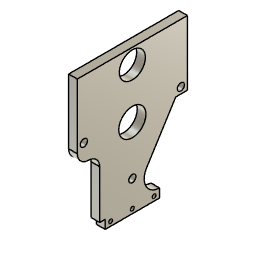
[J,L]C-578VA Mount (Autodesk Fusion 360 design; units mm, degrees)
Autodesk Fusion 360 part; units mm, degrees
sketch "スケッチ1" plane through (0, 0, 0) normal (1, 0, 0) x (0, 1, 0)
  line L0 (0, 0) -> (-44.6, 0)
  line L1 (0, 0) -> (44.6, 0)
  line L2 (-44.6, 0) -> (-44.6, 5.7)
  line L3 (44.6, 0) -> (44.6, 5.7)
  circle A0 centre (-44.6, 5.7) radius 3
  circle A1 centre (44.6, 5.7) radius 3
  line L4 (0, 0) -> (0, 43.5)
  line L5 (0, 43.5) -> (-11.3, 43.5)
  circle A2 centre (-11.3, 43.5) radius 3
  line L6 (0, 0) -> (0, -45)
  circle A3 centre (0, -45) radius 3
  circle A4 centre (-11.3, 43.5) radius 6
  circle A5 centre (-44.6, 5.7) radius 6
  circle A6 centre (44.6, 5.7) radius 6
  circle A7 centre (0, -45) radius 6
  line L7 (50.6, -51) -> (-50.6, -51)
  line L8 (-50.6, -51) -> (-50.6, 51)
  line L9 (-50.6, 51) -> (50.6, 51)
  line L10 (50.6, 51) -> (50.6, -51)
  line L11 (50.6, -51) -> (-50.6, 51) construction
  line L12 (-50.6, -51) -> (50.6, 51) construction
  circle A8 centre (0, 0) radius 10.5
  line L13 (44.6, 5.7) -> (0, -45)
  line L14 (44.6, 5.7) -> (50.6, 5.7) construction
  line L15 (0, -45) -> (4.505, -48.963)
  line L16 (44.6, 5.7) -> (49.105, 1.737)
  line L17 (0, -45) -> (6, -45)
  line L18 (44.6, 5.7) -> (44.6, -0.3)
  dimension "d1" = 44.6
  dimension "d2" = 44.6
  dimension "d3" = 5.7
  dimension "d4" = 5.7
  dimension "d5" = 6
  dimension "d6" = 6
  dimension "d7" = 43.5
  dimension "d8" = 11.3
  dimension "d9" = 6
  dimension "d10" = 45
  dimension "d11" = 6
  dimension "d12" = 12
  dimension "d13" = 12
  dimension "d14" = 12
  dimension "d15" = 12
  dimension "d16" = 101.2
  dimension "d17" = 102
  dimension "d20" = 21
  constraint coincident L0.start L1.start
  constraint horizontal L0
  constraint parallel L0 L1
  constraint perpendicular L0 L2
  constraint perpendicular L1 L3
  constraint coincident L2.end A0.centre
  constraint coincident L3.end A1.centre
  constraint perpendicular L1 L4
  constraint perpendicular L4 L5
  constraint coincident L5.end A2.centre
  constraint perpendicular L1 L6
  constraint coincident L6.end A3.centre
  constraint concentric A2 A4
  constraint concentric A0 A5
  constraint concentric A1 A6
  constraint concentric A3 A7
  constraint horizontal L7
  constraint perpendicular L7 L8
  constraint parallel L7 L9
  constraint parallel L8 L10
  constraint coincident L11 L0.start
  constraint coincident L12 L0.start
  constraint horizontal L14
  constraint coincident A7 L15.end
  constraint perpendicular L13 L15
  constraint coincident A6 L16.end
  constraint perpendicular L13 L16
  constraint coincident A7 L17.end
  constraint perpendicular L6 L17
  constraint coincident A6 L18.end
  constraint perpendicular L14 L18
  measures "d1" distance of L0.start L0.end
  measures "d2" distance of L0.start L1.end
  measures "d3" distance of L0.end L2.end
  measures "d4" distance of L1.end L3.end
  measures "d5" diameter of A0
  measures "d6" diameter of A1
  measures "d7" distance of L0.start L4.end
  measures "d8" distance of L4.end L5.end
  measures "d9" diameter of A2
  measures "d10" distance of L0.start L6.end
  measures "d11" diameter of A3
  measures "d12" diameter of A4
  measures "d13" diameter of A5
  measures "d14" diameter of A6
  measures "d15" diameter of A7
  measures "d16" distance of L8.end L9.end
  measures "d17" distance of L7.end L8.end
  measures "d20" diameter of A8
extrude "押し出し1" add sketch "スケッチ1" along normal blind 8 contours L0 L6 A5 A7 L7 L8 A8 | L0 L1 A5 A6 L8 L9 L10 A8 L13 | L1 L6 A7 A8 L13 | A5 | L6 A3 A7 L13 | L6 A3 A7 L15 | L1 L3 A1 A6 L13 L18 | L1 A6 L18 | A1 A6 L13 L16 | A3 A7 L13 L17 | L3 A1 A6 L16 L18 | A3 A7 L15 L17 | A4
sketch "スケッチ2" plane through (0, 0, -51) normal (0, 0, -1) x (1, 0, 0)
  line L0 (0, 50.6) -> (0, 0)
  line L1 (0, 0) -> (8, 0)
  line L2 (8, 0) -> (8, 50.6)
  line L3 (8, 50.6) -> (0, 50.6)
  line L4 (0, 50.6) -> (8, 50.6)
  line L5 (8, 50.6) -> (8, 0.6)
  line L6 (8, 0.6) -> (0, 0.6)
  line L7 (0, 0.6) -> (0, 50.6)
  dimension "d22" = 50
  constraint horizontal L4
  constraint vertical L5
  constraint horizontal L6
  constraint vertical L7
  constraint coincident L0.start L3.end
  measures "d22" distance of L0.start L6.end
extrude "押し出し2" add sketch "スケッチ2" along normal blind 18 contours L0 L2 L3 L4 L5 L6 L7
sketch "スケッチ3" plane through (0, 0, 0) normal (-1, 0, 0) x (0, -1, 0)
  circle A0 centre (11.3, 43.5) radius 3
  circle A1 centre (44.6, 5.7) radius 3
  circle A2 centre (0, 0) radius 10.5
  circle A3 centre (-44.6, 5.7) radius 3
  circle A4 centre (0, -45) radius 3
  arc A5 (-3.963, -40.495) -> (0, -51) centre (0, -45) ccw
  line L0 (0, -51) -> (0.6, -51)
  line L1 (0.6, -51) -> (0.6, -69)
  line L2 (0.6, -69) -> (50.6, -69)
  line L3 (50.6, -69) -> (50.6, 51)
  line L4 (50.6, 51) -> (-50.6, 51)
  line L5 (-50.6, 51) -> (-50.6, 5.7)
  arc A6 (-50.6, 5.7) -> (-40.637, 1.195) centre (-44.6, 5.7) ccw
  line L6 (-40.637, 1.195) -> (-3.963, -40.495)
  circle A7 centre (0, 0) radius 23.5
  dimension "d25" = 47
  constraint coincident A2.centre A7.centre
  measures "d25" diameter of A7
extrude "押し出し3" cut sketch "スケッチ3" against normal blind 8 contours A7
extrude "押し出し4" add 1 faces at (2.6667, -17.2667, -69) along direction (0, 0, -1) blind 4
box "直方体プリミティブ1" cut length 8 width 8 height -25.6 placed x (0, 0, 1) y (-1, 0, 0) z (0, -1, 0) at (8, -50.6, -73)
box "直方体プリミティブ2" add length 8 width 8 height 25.6 placed x (0, 0, 1) y (1, 0, 0) z (0, 1, 0) at (0, -0.6, -73)
sketch "スケッチ7" plane through (0, 0, 0) normal (-1, 0, 0) x (0, -1, 0)
  line L0 (25, -73) -> (25, -65)
  line L1 (25, -65) -> (50.6, -65)
  line L2 (50.6, -65) -> (50.6, 51)
  line L3 (50.6, 51) -> (-50.6, 51)
  line L4 (-50.6, 51) -> (-50.6, 5.7)
  arc A0 (-50.6, 5.7) -> (-40.637, 1.195) centre (-44.6, 5.7) ccw
  line L5 (-40.637, 1.195) -> (-3.963, -40.495)
  arc A1 (-3.963, -40.495) -> (0, -51) centre (0, -45) ccw
  line L6 (0, -51) -> (0.6, -51)
  line L7 (0.6, -51) -> (0.6, -65)
  line L8 (0.6, -65) -> (-25, -65)
  line L9 (-25, -65) -> (-25, -73)
  line L10 (-25, -73) -> (25, -73)
  circle A2 centre (0, -45) radius 3
  circle A3 centre (-44.6, 5.7) radius 3
  circle A4 centre (44.6, 5.7) radius 3
  circle A5 centre (11.3, 43.5) radius 3
  circle A6 centre (0, 0) radius 23.5
  line L11 (25, -65) -> (30, -65)
  line L12 (0, 0) -> (0, -23.5)
  line L13 (0, -23.5) -> (50.6, -23.5)
  line L14 (30, -65) -> (30, -23.5)
  dimension "d48" = 5
  constraint coincident L0.end L1.start
  constraint perpendicular L0 L11
  constraint coincident A6.centre L12.start
  constraint coincident A6 L12.end
  constraint vertical L12
  constraint coincident L2 L13.end
  constraint tangent A6 L13
  constraint coincident L13 L14.end
  constraint perpendicular L13 L14
  measures "d48" distance of L0.end L11.end
extrude "押し出し6" cut sketch "スケッチ7" against normal blind 8 contours L1 L2 L13 L14
extrude "押し出し7" cut 1 faces at (2.6667, -36.8667, -23.5) along direction (0, 0, 1) blind 5
sketch "スケッチ8" plane through (8, 0, 0) normal (1, 0, 0) x (0, 1, 0)
  line L0 (-50.6, -18.5) -> (-30, -18.5)
  line L1 (-30, -18.5) -> (-30, -65)
  line L2 (-30, -65) -> (-25, -65)
  line L3 (-25, -65) -> (-25, -73)
  line L4 (-25, -73) -> (25, -73)
  line L5 (25, -73) -> (25, -65)
  line L6 (25, -65) -> (-0.6, -65)
  line L7 (-0.6, -65) -> (-0.6, -51)
  line L8 (-0.6, -51) -> (0, -51)
  arc A0 (0, -51) -> (3.963, -40.495) centre (0, -45) ccw
  line L9 (3.963, -40.495) -> (40.637, 1.195)
  arc A1 (40.637, 1.195) -> (50.6, 5.7) centre (44.6, 5.7) ccw
  line L10 (50.6, 5.7) -> (50.6, 51)
  line L11 (50.6, 51) -> (-50.6, 51)
  line L12 (-50.6, 51) -> (-50.6, -18.5)
  circle A2 centre (0, -45) radius 3
  circle A3 centre (44.6, 5.7) radius 3
  circle A4 centre (-44.6, 5.7) radius 3
  circle A5 centre (-11.3, 43.5) radius 3
  circle A6 centre (0, 0) radius 23.5
  line L13 (40.637, 1.195) -> (-0.6, -65)
  constraint coincident L9.end A1.start
  constraint coincident L6.end L7.start
extrude "押し出し8" add sketch "スケッチ8" against normal blind 8 contours L7 L8 A0 L9 L13
fillet "フィレット1" radius 14.3 1 edges at (4, -0.6, -65)
fillet "フィレット2" radius 10.3 1 edges at (4, -50.6, -18.5)
fillet "フィレット3" radius 10.3 1 edges at (4, -30, -18.5)
sketch "スケッチ9" plane through (8, 0, 0) normal (1, 0, 0) x (0, 1, 0)
  arc A0 (-50.6, -8.2) -> (-40.3, -18.5) centre (-40.3, -8.2) ccw
  arc A1 (-30, -28.8) -> (-40.3, -18.5) centre (-40.3, -28.8) ccw
  line L0 (-30, -28.8) -> (-30, -65)
  line L1 (-30, -65) -> (-25, -65)
  line L2 (-25, -65) -> (-25, -73)
  line L3 (-25, -73) -> (25, -73)
  line L4 (25, -73) -> (25, -65)
  arc A2 (13.0182, -43.1397) -> (25, -65) centre (25.1557, -50.7008) ccw
  line L5 (13.0182, -43.1397) -> (40.637, 1.195)
  arc A3 (40.637, 1.195) -> (50.6, 5.7) centre (44.6, 5.7) ccw
  line L6 (50.6, 5.7) -> (50.6, 51)
  line L7 (50.6, 51) -> (-50.6, 51)
  line L8 (-50.6, 51) -> (-50.6, -8.2)
  circle A4 centre (0, -45) radius 3
  circle A5 centre (44.6, 5.7) radius 3
  circle A6 centre (-44.6, 5.7) radius 3
  circle A7 centre (-11.3, 43.5) radius 3
  circle A8 centre (0, 0) radius 23.5
  line L9 (-25, -69) -> (25, -69)
  line L10 (0, -69) -> (20, -69)
  line L11 (0, -69) -> (-20, -69)
  circle A9 centre (0, -69) radius 1.7
  circle A10 centre (-20, -69) radius 1.7
  circle A11 centre (20, -69) radius 1.7
  dimension "d61" = 20
  dimension "d62" = 20
  dimension "d63" = 3.4
  dimension "d64" = 3.4
  dimension "d65" = 3.4
  constraint midpoint L2 L9.start
  constraint midpoint L4 L9.end
  constraint midpoint L9 L10.start
  constraint perpendicular L4 L10
  constraint parallel L9 L11
  constraint coincident L10.start L11.start
  constraint coincident L11.end A10.centre
  constraint coincident L10.end A11.centre
  measures "d61" distance of L10.start L10.end
  measures "d62" distance of L10.start L11.end
  measures "d63" diameter of A9
  measures "d64" diameter of A10
  measures "d65" diameter of A11
extrude "押し出し9" cut sketch "スケッチ9" against normal blind 8 contours L9 L11 A10 | L9 L11 A10 | L9 L10 L11 A9 | L9 L10 L11 A9 | L9 L10 A11 | L9 L10 A11
sketch "スケッチ10" plane through (8, 0, 0) normal (1, 0, 0) x (0, 1, 0)
  circle A0 centre (20, -69) radius 1.7
  circle A1 centre (0, -69) radius 1.7
  circle A2 centre (-20, -69) radius 1.7
  arc A3 (-50.6, -8.2) -> (-40.3, -18.5) centre (-40.3, -8.2) ccw
  arc A4 (-30, -28.8) -> (-40.3, -18.5) centre (-40.3, -28.8) ccw
  line L0 (-30, -28.8) -> (-30, -65)
  line L1 (-30, -65) -> (-25, -65)
  line L2 (-25, -65) -> (-25, -73)
  line L3 (-25, -73) -> (25, -73)
  line L4 (25, -73) -> (25, -65)
  arc A5 (13.0182, -43.1397) -> (25, -65) centre (25.1557, -50.7008) ccw
  line L5 (13.0182, -43.1397) -> (40.637, 1.195)
  arc A6 (40.637, 1.195) -> (50.6, 5.7) centre (44.6, 5.7) ccw
  line L6 (50.6, 5.7) -> (50.6, 51)
  line L7 (50.6, 51) -> (-50.6, 51)
  line L8 (-50.6, 51) -> (-50.6, -8.2)
  circle A7 centre (0, -45) radius 3
  circle A8 centre (44.6, 5.7) radius 3
  circle A9 centre (-44.6, 5.7) radius 3
  circle A10 centre (-11.3, 43.5) radius 3
  circle A11 centre (0, 0) radius 23.5
  line L9 (0, 0) -> (0, 45.5)
  circle A12 centre (0, 45.5) radius 12
  line L10 (-50.6, 51) -> (0, 51)
  line L11 (0, 51) -> (0, 57.5)
  line L12 (0, 57.5) -> (-50.6, 57.5)
  line L13 (-50.6, 57.5) -> (-50.6, 51)
  line L14 (50.6, 51) -> (0, 51)
  line L15 (0, 51) -> (0, 57.5)
  line L16 (0, 57.5) -> (50.6, 57.5)
  line L17 (50.6, 57.5) -> (50.6, 51)
  line L18 (-50.6, 57.5) -> (50.6, 57.5)
  line L19 (50.6, 57.5) -> (50.6, 59.5)
  line L20 (50.6, 59.5) -> (-50.6, 59.5)
  line L21 (-50.6, 59.5) -> (-50.6, 57.5)
  dimension "d68" = 45.5
  dimension "d69" = 24
  dimension "d72" = 2
  constraint coincident A11.centre L9.start
  constraint vertical L9
  constraint coincident L9.end A12.centre
  constraint horizontal L10
  constraint vertical L11
  constraint horizontal L12
  constraint vertical L13
  constraint coincident A12 L11.end
  constraint coincident L7.end L8.start
  constraint horizontal L14
  constraint vertical L15
  constraint horizontal L16
  constraint vertical L17
  constraint coincident L6.end L7.start
  constraint horizontal L18
  constraint vertical L19
  constraint horizontal L20
  constraint vertical L21
  measures "d68" distance of A11.centre L9.end
  measures "d69" diameter of A12
  measures "d72" distance of L12.end L20.end
extrude "押し出し11" add sketch "スケッチ10" against normal blind 8 contours L7 A12 L10 L12 L13 L18 | L12 L16 L18 L19 L20 L21 | L7 A12 L14 L16 L17 L18
extrude "押し出し12" cut sketch "スケッチ10" against normal blind 8 contours L7 A10 A12 L10 L14
extrude "押し出し13" add sketch "スケッチ10" against normal blind 8 contours A10 A12 picked at (-12.6459, 44.2666)
sketch "スケッチ11" plane through (8, 0, 0) normal (1, 0, 0) x (0, 1, 0)
  circle A0 centre (0, 45.5) radius 12
  line L0 (-50.6, 59.5) -> (-50.6, -8.2)
  arc A1 (-50.6, -8.2) -> (-40.3, -18.5) centre (-40.3, -8.2) ccw
  arc A2 (-30, -28.8) -> (-40.3, -18.5) centre (-40.3, -28.8) ccw
  line L1 (-30, -28.8) -> (-30, -65)
  line L2 (-30, -65) -> (-25, -65)
  line L3 (-25, -65) -> (-25, -73)
  line L4 (-25, -73) -> (25, -73)
  line L5 (25, -73) -> (25, -65)
  arc A3 (13.0182, -43.1397) -> (25, -65) centre (25.1557, -50.7008) ccw
  line L6 (13.0182, -43.1397) -> (40.637, 1.195)
  arc A4 (40.637, 1.195) -> (50.6, 5.7) centre (44.6, 5.7) ccw
  line L7 (50.6, 5.7) -> (50.6, 59.5)
  line L8 (50.6, 59.5) -> (-50.6, 59.5)
  circle A5 centre (20, -69) radius 1.7
  circle A6 centre (0, -69) radius 1.7
  circle A7 centre (-20, -69) radius 1.7
  circle A8 centre (0, -45) radius 3
  circle A9 centre (44.6, 5.7) radius 3
  circle A10 centre (-44.6, 5.7) radius 3
  circle A11 centre (0, 0) radius 23.5
  circle A12 centre (0, 0) radius 13
  dimension "d79" = 26
  constraint coincident A11.centre A12.centre
  measures "d79" diameter of A12
extrude "押し出し14" add sketch "スケッチ11" against normal blind 8 contours A11
sketch "スケッチ12" plane through (8, 0, 0) normal (1, 0, 0) x (0, 1, 0)
  circle A0 centre (0, 0) radius 13
  circle A1 centre (0, 45.5) radius 12
  line L0 (-50.6, 59.5) -> (-50.6, -8.2)
  arc A2 (-50.6, -8.2) -> (-40.3, -18.5) centre (-40.3, -8.2) ccw
  arc A3 (-30, -28.8) -> (-40.3, -18.5) centre (-40.3, -28.8) ccw
  line L1 (-30, -28.8) -> (-30, -65)
  line L2 (-30, -65) -> (-25, -65)
  line L3 (-25, -65) -> (-25, -73)
  line L4 (-25, -73) -> (25, -73)
  line L5 (25, -73) -> (25, -65)
  arc A4 (13.0182, -43.1397) -> (25, -65) centre (25.1557, -50.7008) ccw
  line L6 (13.0182, -43.1397) -> (40.637, 1.195)
  arc A5 (40.637, 1.195) -> (50.6, 5.7) centre (44.6, 5.7) ccw
  line L7 (50.6, 5.7) -> (50.6, 59.5)
  line L8 (50.6, 59.5) -> (-50.6, 59.5)
  circle A6 centre (20, -69) radius 1.7
  circle A7 centre (0, -69) radius 1.7
  circle A8 centre (-20, -69) radius 1.7
  circle A9 centre (0, -45) radius 3
  circle A10 centre (44.6, 5.7) radius 3
  circle A11 centre (-44.6, 5.7) radius 3
  line L9 (44.6, 5.7) -> (44.6, -0.3)
  line L10 (44.6, -0.3) -> (39.7057, -0.3)
  constraint coincident A5.centre A10.centre
  constraint coincident A5 L9.end
  constraint vertical L9
  constraint coincident L6 L10.end
  constraint tangent A5 L10
extrude "押し出し15" add sketch "スケッチ12" against normal blind 8 contours L6 A5 L10
sketch "スケッチ13" plane through (8, 0, 0) normal (1, 0, 0) x (0, 1, 0)
  circle A0 centre (0, 0) radius 13
  circle A1 centre (0, 45.5) radius 12
  line L0 (-50.6, 59.5) -> (-50.6, -8.2)
  arc A2 (-50.6, -8.2) -> (-40.3, -18.5) centre (-40.3, -8.2) ccw
  arc A3 (-30, -28.8) -> (-40.3, -18.5) centre (-40.3, -28.8) ccw
  line L1 (-30, -28.8) -> (-30, -65)
  line L2 (-30, -65) -> (-25, -65)
  line L3 (-25, -65) -> (-25, -73)
  line L4 (-25, -73) -> (25, -73)
  line L5 (25, -73) -> (25, -65)
  arc A4 (13.0182, -43.1397) -> (25, -65) centre (25.1557, -50.7008) ccw
  line L6 (13.0182, -43.1397) -> (39.7057, -0.3)
  line L7 (39.7057, -0.3) -> (44.6, -0.3)
  arc A5 (44.6, -0.3) -> (50.6, 5.7) centre (44.6, 5.7) ccw
  line L8 (50.6, 5.7) -> (50.6, 59.5)
  line L9 (50.6, 59.5) -> (-50.6, 59.5)
  circle A6 centre (20, -69) radius 1.7
  circle A7 centre (0, -69) radius 1.7
  circle A8 centre (-20, -69) radius 1.7
  circle A9 centre (0, -45) radius 3
  circle A10 centre (44.6, 5.7) radius 3
  circle A11 centre (-44.6, 5.7) radius 3
  line L10 (0, 0) -> (-50.6, 0)
  line L11 (44.6, 5.7) -> (44.6, 0)
  line L12 (44.6, 0) -> (0, 0)
  line L13 (50.6, 5.7) -> (44.6, 5.7)
  line L14 (44.6, 5.7) -> (44.6, 0)
  line L15 (44.6, 0) -> (50.6, 0)
  line L16 (50.6, 0) -> (50.6, 5.7)
  constraint coincident A0.centre L10.start
  constraint coincident L0 L10.end
  constraint perpendicular L0 L10
  constraint coincident A5.centre A10.centre
  constraint perpendicular L10 L11
  constraint perpendicular L11 L12
  constraint horizontal L13
  constraint vertical L14
  constraint horizontal L15
  constraint vertical L16
  constraint coincident A5.end L8.start
extrude "押し出し17" add sketch "スケッチ13" against normal blind 8 contours A5 L15 L16
sketch "スケッチ14" plane through (8, 0, 0) normal (1, 0, 0) x (0, 1, 0)
  circle A0 centre (0, 0) radius 13
  circle A1 centre (0, 45.5) radius 12
  line L0 (-50.6, 59.5) -> (-50.6, -8.2)
  arc A2 (-50.6, -8.2) -> (-40.3, -18.5) centre (-40.3, -8.2) ccw
  arc A3 (-30, -28.8) -> (-40.3, -18.5) centre (-40.3, -28.8) ccw
  line L1 (-30, -28.8) -> (-30, -65)
  line L2 (-30, -65) -> (-25, -65)
  line L3 (-25, -65) -> (-25, -73)
  line L4 (-25, -73) -> (25, -73)
  line L5 (25, -73) -> (25, -65)
  arc A4 (13.0182, -43.1397) -> (25, -65) centre (25.1557, -50.7008) ccw
  line L6 (13.0182, -43.1397) -> (39.7057, -0.3)
  line L7 (39.7057, -0.3) -> (44.6, -0.3)
  arc A5 (44.6, -0.3) -> (46.4735, 0) centre (44.6, 5.7) ccw
  line L8 (46.4735, 0) -> (50.6, 0)
  line L9 (50.6, 0) -> (50.6, 59.5)
  line L10 (50.6, 59.5) -> (-50.6, 59.5)
  circle A6 centre (20, -69) radius 1.7
  circle A7 centre (0, -69) radius 1.7
  circle A8 centre (-20, -69) radius 1.7
  circle A9 centre (0, -45) radius 3
  circle A10 centre (44.6, 5.7) radius 3
  circle A11 centre (-44.6, 5.7) radius 3
  line L11 (0, 0) -> (46.4735, 0)
  line L12 (39.7057, -0.3) -> (39.8926, 0)
  constraint coincident A0.centre L11.start
  constraint coincident A5.end L8.start
  constraint coincident L6.end L7.start
  constraint coincident L11 L12.end
  constraint parallel L6 L12
extrude "押し出し18" cut sketch "スケッチ14" against normal blind 8 contours L7 A5 L11 L12
sketch "スケッチ15" plane through (8, 0, 0) normal (1, 0, 0) x (0, 1, 0)
  line L0 (39.8926, 0) -> (50.6, 0)
  line L1 (50.6, 0) -> (50.6, 59.5)
  line L2 (50.6, 59.5) -> (-50.6, 59.5)
  line L3 (-50.6, 59.5) -> (-50.6, -8.2)
  arc A0 (-50.6, -8.2) -> (-40.3, -18.5) centre (-40.3, -8.2) ccw
  arc A1 (-30, -28.8) -> (-40.3, -18.5) centre (-40.3, -28.8) ccw
  line L4 (-30, -28.8) -> (-30, -65)
  line L5 (-30, -65) -> (-25, -65)
  line L6 (-25, -65) -> (-25, -73)
  line L7 (-25, -73) -> (25, -73)
  line L8 (25, -73) -> (25, -65)
  arc A2 (13.0182, -43.1397) -> (25, -65) centre (25.1557, -50.7008) ccw
  line L9 (13.0182, -43.1397) -> (39.8926, 0)
  circle A3 centre (0, 0) radius 13
  circle A4 centre (0, 45.5) radius 12
  circle A5 centre (20, -69) radius 1.7
  circle A6 centre (0, -69) radius 1.7
  circle A7 centre (-20, -69) radius 1.7
  circle A8 centre (0, -45) radius 3
  circle A9 centre (44.6, 5.7) radius 3
  circle A10 centre (-44.6, 5.7) radius 3
  line L10 (0, 0) -> (-50.6, 0)
  line L11 (-40.3, -18.5) -> (-40.3, 0)
  circle A11 centre (-40.3, 0) radius 10.3
  line L12 (-40.3, -10.3) -> (-30, -10.3)
  line L13 (-30, -10.3) -> (-30, -20.6)
  line L14 (-30, -20.6) -> (-40.3, -20.6)
  line L15 (-40.3, -20.6) -> (-40.3, -10.3)
  circle A12 centre (-40.3, -20.6) radius 10.3
  line L16 (-30, -20.6) -> (-30, -28.8)
  dimension "d93" = 10.3
  dimension "d94" = 10.3
  constraint coincident A3.centre L10.start
  constraint coincident L3 L10.end
  constraint perpendicular L3 L10
  constraint coincident A0.end A1.end
  constraint coincident L10 L11.end
  constraint perpendicular L10 L11
  constraint coincident L11.end A11.centre
  constraint coincident L10.end A11
  constraint horizontal L12
  constraint vertical L13
  constraint horizontal L14
  constraint vertical L15
  constraint coincident A11 L12.start
  constraint coincident L11 L12.start
  constraint coincident L14.end L15.start
  constraint coincident L12.start A12
  constraint coincident A1.start L4.start
  measures "d93" distance of L12.start L12.end
  measures "d94" distance of L12.start L14.end
extrude "押し出し19" cut sketch "スケッチ15" against normal blind 8 contours L3 A0 A11 A12 | A1 L11 L14 L15 A12 | A0 L11 L15 A12 | A1 L14 A12 | A1 A12 L16
sketch "スケッチ16" plane through (8, 0, 0) normal (1, 0, 0) x (0, 1, 0)
  circle A0 centre (-44.6, 5.7) radius 3
  circle A1 centre (44.6, 5.7) radius 3
  circle A2 centre (0, -45) radius 3
  circle A3 centre (-20, -69) radius 1.7
  circle A4 centre (0, -69) radius 1.7
  circle A5 centre (20, -69) radius 1.7
  circle A6 centre (0, 45.5) radius 12
  circle A7 centre (0, 0) radius 13
  arc A8 (-50.6, 0) -> (-40.3, -10.3) centre (-40.3, 0) ccw
  arc A9 (-30, -20.6) -> (-40.3, -10.3) centre (-40.3, -20.6) ccw
  line L0 (-30, -20.6) -> (-30, -65)
  line L1 (-30, -65) -> (-25, -65)
  line L2 (-25, -65) -> (-25, -73)
  line L3 (-25, -73) -> (25, -73)
  line L4 (25, -73) -> (25, -65)
  arc A10 (13.0182, -43.1397) -> (25, -65) centre (25.1557, -50.7008) ccw
  line L5 (13.0182, -43.1397) -> (39.8926, 0)
  line L6 (39.8926, 0) -> (50.6, 0)
  line L7 (50.6, 0) -> (50.6, 59.5)
  line L8 (50.6, 59.5) -> (-50.6, 59.5)
  line L9 (-50.6, 59.5) -> (-50.6, 0)
  circle A11 centre (-44.6, 5.7) radius 3.3
  circle A12 centre (44.6, 5.7) radius 3.3
  circle A13 centre (0, -45) radius 3.3
  circle A14 centre (0, 0) radius 13.5
  dimension "d97" = 6.6
  dimension "d98" = 6.6
  dimension "d99" = 6.6
  dimension "d100" = 27
  constraint concentric A0 A11
  constraint concentric A1 A12
  constraint concentric A2 A13
  constraint concentric A7 A14
  measures "d97" diameter of A11
  measures "d98" diameter of A12
  measures "d99" diameter of A13
  measures "d100" diameter of A14
extrude "押し出し20" cut sketch "スケッチ16" against normal blind 8 contours A11 | A12 | A13
sketch "スケッチ17" plane through (8, 0, 0) normal (1, 0, 0) x (0, 1, 0)
  circle A0 centre (44.6, 5.7) radius 3.3
  circle A1 centre (-44.6, 5.7) radius 3.3
  circle A2 centre (0, -45) radius 3.3
  circle A3 centre (-20, -69) radius 1.7
  circle A4 centre (0, -69) radius 1.7
  circle A5 centre (20, -69) radius 1.7
  circle A6 centre (0, 45.5) radius 12
  circle A7 centre (0, 0) radius 13
  arc A8 (-50.6, 0) -> (-40.3, -10.3) centre (-40.3, 0) ccw
  arc A9 (-30, -20.6) -> (-40.3, -10.3) centre (-40.3, -20.6) ccw
  line L0 (-30, -20.6) -> (-30, -65)
  line L1 (-30, -65) -> (-25, -65)
  line L2 (-25, -65) -> (-25, -73)
  line L3 (-25, -73) -> (25, -73)
  line L4 (25, -73) -> (25, -65)
  arc A10 (13.0182, -43.1397) -> (25, -65) centre (25.1557, -50.7008) ccw
  line L5 (13.0182, -43.1397) -> (39.8926, 0)
  line L6 (39.8926, 0) -> (50.6, 0)
  line L7 (50.6, 0) -> (50.6, 59.5)
  line L8 (50.6, 59.5) -> (-50.6, 59.5)
  line L9 (-50.6, 59.5) -> (-50.6, 0)
  circle A11 centre (0, 0) radius 12.5
  dimension "d103" = 25
  constraint concentric A7 A11
  measures "d103" diameter of A11
extrude "押し出し21" add sketch "スケッチ17" against normal blind 8 contours A7
equation "d16 = 44.6 mm + 44.6 mm + 12 mm"
equation "d17 = 45 mm + 45 mm + 12 mm"
